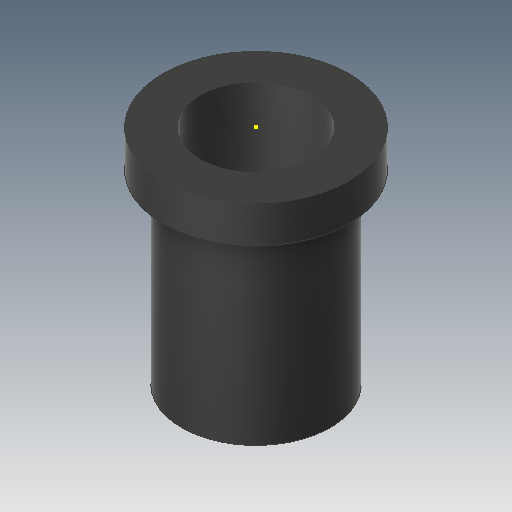
# Autodesk Inventor part: DiffusionModule
Saved by Autodesk Inventor 2020.3 (Build 243373000, 373)
## iProperties
Created: 2021-08-11
Part Number: DiffusionModule
Material: ABS Plastic
Document SubType Name: Modeling
Designer: justi
Density: 1.06 g/cm^3
Appearance: Smooth - Black
Mass: 5.71193 g
Surface Area: 43.1655 cm^2
Volume: 5.38862 cm^3
Author: justi
Autodesk Inventor part; units mm, degrees
ref_plane "YZ Plane" through (0, 0, 0) normal (1, 0, 0) x (0, 1, 0)
ref_plane "XZ Plane" through (0, 0, 0) normal (0, 1, 0) x (-1, 0, 0)
ref_plane "XY Plane" through (0, 0, 0) normal (0, 0, 1) x (1, 0, 0)
sketch "Sketch1" plane through (0, 0, 0) normal (0, 1, 0) x (-1, 0, 0)
  circle A0 centre (0, 0) radius 10
  dimension "d0" = 20
  constraints: 1 centre point, 1 coincident
  measures "d0" diameter of A0
extrude "Extrusion1" add sketch "Sketch1" along normal blind 30
sketch "Sketch2" plane through (0, 30, 0) normal (0, 1, 0) x (1, 0, 0)
  circle A0 centre (0, 0) radius 12.5
  dimension "d3" = 25
  constraints: 1 centre point, 1 coincident
  measures "d3" diameter of A0
extrude "Extrusion2" add sketch "Sketch2" against normal blind 5
sketch "Sketch3" plane through (0, 30, 0) normal (0, 1, 0) x (1, 0, 0)
  circle A0 centre (0, 0) radius 7.5
  dimension "d7" = 15
  constraints: 1 centre point, 1 coincident
  measures "d7" diameter of A0
extrude "Extrusion3" cut sketch "Sketch3" against normal blind 27
sketch "Sketch5" plane through (0, 0, 0) normal (0, -1, 0) x (1, 0, 0)
  circle A0 centre (0, 0) radius 5 construction
  circle A1 centre (0, 5) radius 1.5
  circle A2 centre (0, 0) radius 5 construction
  circle A3 centre (-4.3301, 2.5) radius 1.5
  circle A4 centre (0, 0) radius 5 construction
  circle A5 centre (-4.3301, -2.5) radius 1.5
  circle A6 centre (0, 0) radius 5 construction
  circle A7 centre (0, -5) radius 1.5
  circle A8 centre (0, 0) radius 5 construction
  circle A9 centre (4.3301, -2.5) radius 1.5
  circle A10 centre (0, 0) radius 5 construction
  circle A11 centre (4.3301, 2.5) radius 1.5
  circle A12 centre (0, 0) radius 1.5
  dimension "d32" = 10
  dimension "d33" = 3
  dimension "d36" = 360
  dimension "d38" = 3
  constraints: 7 centre point, 2 coincident, 2 vertical alignment, 41 other
  measures "d33" diameter of A1
  measures "d38" diameter of A12
extrude "Extrusion6" cut sketch "Sketch5" against normal blind 10
sketch "Sketch6" plane through (0, 30, 0) normal (0, 1, 0) x (1, 0, 0)
  point P0 (0, 0)
body "Solid1"
